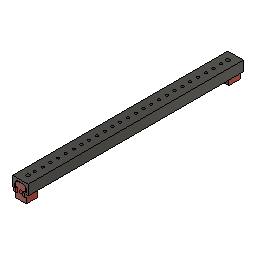
5_Assembly_Electro_support v5 (Autodesk Fusion 360 archive; units mm, degrees)
design "Support CI"
Autodesk Fusion 360 part; units mm, degrees
sketch "Sketch1" plane through (0, 0, 0) normal (0, 0, 1) x (1, 0, 0) in component "Support Electo"
  line L0 (138.5, -10) -> (-138.5, -10)
  line L1 (-138.5, -10) -> (-138.5, 10)
  line L2 (-138.5, 10) -> (138.5, 10)
  line L3 (138.5, 10) -> (138.5, -10)
  line L4 (138.5, -10) -> (-138.5, 10) construction
  line L5 (-138.5, -10) -> (138.5, 10) construction
  line L6 (138.5, -10) -> (138.5, 10)
  circle A0 centre (0, 0) radius 1.6
  circle A1 centre (-120, 0) radius 1.6
  circle A2 centre (-110, 0) radius 1.6
  circle A3 centre (-100, 0) radius 1.6
  circle A4 centre (-90, 0) radius 1.6
  circle A5 centre (-80, 0) radius 1.6
  circle A6 centre (-70, 0) radius 1.6
  circle A7 centre (-60, 0) radius 1.6
  circle A8 centre (-50, 0) radius 1.6
  circle A9 centre (-40, 0) radius 1.6
  circle A10 centre (-30, 0) radius 1.6
  circle A11 centre (-20, 0) radius 1.6
  circle A12 centre (-10, 0) radius 1.6
  circle A13 centre (10, 0) radius 1.6
  circle A14 centre (20, 0) radius 1.6
  circle A15 centre (30, 0) radius 1.6
  circle A16 centre (40, 0) radius 1.6
  circle A17 centre (50, 0) radius 1.6
  circle A18 centre (60, 0) radius 1.6
  circle A19 centre (70, 0) radius 1.6
  circle A20 centre (80, 0) radius 1.6
  circle A21 centre (90, 0) radius 1.6
  circle A22 centre (100, 0) radius 1.6
  circle A23 centre (110, 0) radius 1.6
  circle A24 centre (120, 0) radius 1.6
  line L7 (-138.5, 10) -> (138.5, 10)
  line L8 (138.5, 10) -> (138.5, 7)
  line L9 (138.5, 7) -> (-138.5, 7)
  line L10 (-138.5, 7) -> (-138.5, 10)
  line L11 (-138.5, -7) -> (138.5, -7)
  line L12 (138.5, -7) -> (138.5, -10)
  line L13 (138.5, -10) -> (-138.5, -10)
  line L14 (-138.5, -10) -> (-138.5, -7)
  line L15 (-138.5, -10) -> (-138.5, -7)
  line L16 (-138.5, 7) -> (-138.5, 10)
  circle A25 centre (-128.5, 0) radius 2.25
  circle A26 centre (128.5, 0) radius 2.25
  line L17 (-138.5, 0) -> (138.5, 0) construction
  dimension "d171" = 277
  dimension "d172" = 20
  dimension "d174" = 20
  dimension "d176" = 20
  dimension "d189" = 3.2
  dimension "d192" = 10
  dimension "d193" = 0
  dimension "d194" = 3
  dimension "d195" = 3
  dimension "d225" = 4.5
  dimension "d226" = 10
  dimension "d227" = 4.5
  dimension "d228" = 10
  constraint horizontal L0
  constraint perpendicular L0 L1
  constraint parallel L0 L2
  constraint parallel L1 L3
  constraint coincident L4 A0.centre
  constraint coincident L5 A0.centre
  constraint coincident A0.centre origin
  constraint vertical L15
  constraint vertical L6
  constraint horizontal L7
  constraint vertical L8
  constraint horizontal L9
  constraint vertical L10
  constraint coincident L3 L8.end
  constraint horizontal L11
  constraint vertical L12
  constraint horizontal L13
  constraint vertical L14
  constraint collinear L15 L16
  constraint midpoint L1 L17.start
  constraint midpoint L6 L17.end
  constraint coincident A26.centre L17
  constraint coincident A25.centre L17
  measures "d171" distance of L1.end L2.end
  measures "d172" distance of L0.end L1.end
  measures "d174" distance of L1.end L0.end
  measures "d176" distance of L2.end L0.start
  measures "d189" diameter of A0
  measures "d194" distance of L1.end L9.end
  measures "d195" distance of L11.start L0.end
  measures "d225" diameter of A25
  measures "d226" distance of L1 A25.centre
  measures "d227" diameter of A26
  measures "d228" distance of L6 A26.centre
extrude "Extrude6" add sketch "Sketch1" along normal blind 3 makes body 1 in component "Support Electo"
extrude "Extrude7" add sketch "Sketch1" against normal blind 10 contours L0 L1 L3 L6 L11 L12 L13 L14 L15 | L1 L2 L3 L6 L7 L8 L9 L10 L16 bodies 1 in component "Support Electo"
fillet "Fillet2" radius 4 2 edges at (0, 7, 0) (0, -7, 0) on bodies 1 in component "Support Electo"
sketch "Sketch1 (2)" plane through (0, 4.3249, 0) normal (0, -1, 0) x (1, 0, 0) in component "Equerre"
  line L0 (266.4871, 11.1429) -> (266.4871, 24.1429)
  line L1 (266.4871, 24.1429) -> (246.4871, 24.1429)
  line L2 (246.4871, 24.1429) -> (246.4871, 11.1429)
  line L3 (246.4871, 11.1429) -> (249.4871, 11.1429)
  line L4 (249.4871, 11.1429) -> (249.4871, 17.1429)
  arc A0 (253.4871, 21.1429) -> (249.4871, 17.1429) centre (253.4871, 17.1429) ccw
  line L5 (253.4871, 21.1429) -> (259.4871, 21.1429)
  arc A1 (263.4871, 17.1429) -> (259.4871, 21.1429) centre (259.4871, 17.1429) ccw
  line L6 (263.4871, 17.1429) -> (263.4871, 11.1429)
  line L7 (263.4871, 11.1429) -> (266.4871, 11.1429)
  arc A2 (263.4871, 17.1429) -> (259.4871, 21.1429) centre (259.4871, 17.1429) ccw
  line L8 (263.4871, 17.1429) -> (263.4871, 11.1429)
  line L9 (259.4871, 21.1429) -> (253.4871, 21.1429)
  arc A3 (253.4871, 21.1429) -> (249.4871, 17.1429) centre (253.4871, 17.1429) ccw
  line L10 (249.4871, 17.1429) -> (249.4871, 11.1429)
  line L11 (263.3871, 17.1429) -> (263.3871, 5.9705)
  line L12 (249.5871, 17.1429) -> (249.5871, 5.9705)
  arc A4 (253.4871, 21.0429) -> (249.5871, 17.1429) centre (253.4871, 17.1429) ccw
  line L13 (259.4871, 21.0429) -> (253.4871, 21.0429)
  arc A5 (263.3871, 17.1429) -> (259.4871, 21.0429) centre (259.4871, 17.1429) ccw
  line L14 (263.3871, 5.9705) -> (263.3871, 1.0429)
  line L15 (263.3871, 1.0429) -> (249.5871, 1.0429)
  line L16 (249.5871, 1.0429) -> (249.5871, 5.9705)
  line L17 (249.5871, 10.9429) -> (249.5871, 11.1429)
  line L18 (263.3871, 11.1429) -> (263.3871, 10.9429)
  line L19 (249.4871, 11.1429) -> (249.5871, 11.1429)
  circle A6 centre (256.4871, 11.0429) radius 2.1
  line L20 (249.5871, 11.0429) -> (263.3871, 11.0429) construction
  line L21 (263.3871, 8.0429) -> (249.5871, 8.0429)
  line L22 (249.5871, 8.0429) -> (249.5871, 14.0429)
  line L23 (249.5871, 14.0429) -> (263.3871, 14.0429)
  line L24 (263.3871, 14.0429) -> (263.3871, 8.0429)
  line L25 (263.3871, 8.0429) -> (249.5871, 14.0429) construction
  line L26 (249.5871, 8.0429) -> (263.3871, 14.0429) construction
  line L27 (260.9871, 8.0429) -> (251.9871, 8.0429)
  line L28 (251.9871, 8.0429) -> (251.9871, 14.0429)
  line L29 (251.9871, 14.0429) -> (260.9871, 14.0429)
  line L30 (260.9871, 14.0429) -> (260.9871, 8.0429)
  line L31 (260.9871, 8.0429) -> (251.9871, 14.0429) construction
  line L32 (251.9871, 8.0429) -> (260.9871, 14.0429) construction
  point P0 (256.4871, 11.0429)
  point P1 (256.4871, 11.0429)
  point P2 (256.4871, 11.0429)
  dimension "d268" = 4.2
  dimension "d273" = 20
  dimension "d274" = 0.1
  dimension "d275" = 10
  dimension "d276" = 6
  dimension "d282" = 9
  constraint coincident L3.end L4.start
  constraint vertical L14
  constraint horizontal L15
  constraint vertical L16
  constraint coincident L11.end L14.start
  constraint parallel L17 L18
  constraint coincident L14 L18.start
  constraint parallel L8 L11
  constraint parallel L10 L12
  constraint concentric A3 A4
  constraint parallel L9 L13
  constraint concentric A2 A5
  constraint tangent L13 A5
  constraint tangent L11 A5
  constraint tangent A4 L13
  constraint tangent L12 A4
  constraint coincident P2 P1
  constraint coincident L12 L20.start
  constraint coincident L11 L20.end
  constraint perpendicular L11 L20
  constraint coincident P2 L20
  constraint midpoint P2 L20
  constraint horizontal L21
  constraint perpendicular L21 L22
  constraint parallel L21 L23
  constraint parallel L22 L24
  constraint coincident L11 L21.start
  constraint coincident L25 P2
  constraint coincident L26 P2
  constraint horizontal L27
  constraint perpendicular L27 L28
  constraint parallel L27 L29
  constraint parallel L28 L30
  constraint coincident L31 P2
  constraint coincident L32 P2
  constraint coincident L21 L27.start
  measures "d268" diameter of A6
  measures "d273" distance of L13 L15
  measures "d274" distance of L4 L12
  measures "d275" distance of L15 L20
  measures "d276" distance of L21 L23
  measures "d282" distance of L28.end L29.end
extrude "Extrude1" add sketch "Sketch1 (2)" against normal blind 15 separate body contours L11 L12 A4 L13 A5 L23 L29 | L11 L18 L21 L23 L24 L30 | L21 L23 L27 L28 L29 L30 | L12 L17 L21 L22 L23 L28 | L11 L12 L14 L15 L16 L21 L27 makes body 2 in component "Equerre"
extrude "Extrude3" add sketch "Sketch1 (2)" along normal blind 2 contours L11 L18 L21 L23 L24 L30 | L12 L17 L21 L22 L23 L28 bodies 2 in component "Equerre"
sketch "Sketch2" plane through (0, 0, 21.1429) normal (0, 0, -1) x (1, 0, 0) in component "Equerre"
  line L0 (259.4871, -281.3249) -> (259.4871, -4.3249)
  line L1 (259.4871, -4.3249) -> (253.4871, -4.3249)
  line L2 (253.4871, -4.3249) -> (253.4871, -281.3249)
  line L3 (253.4871, -281.3249) -> (259.4871, -281.3249)
  circle A0 centre (256.4871, -142.8249) radius 1.6
  circle A1 centre (256.4871, -22.8249) radius 1.6
  circle A2 centre (256.4871, -32.8249) radius 1.6
  circle A3 centre (256.4871, -42.8249) radius 1.6
  circle A4 centre (256.4871, -52.8249) radius 1.6
  circle A5 centre (256.4871, -62.8249) radius 1.6
  circle A6 centre (256.4871, -72.8249) radius 1.6
  circle A7 centre (256.4871, -82.8249) radius 1.6
  circle A8 centre (256.4871, -92.8249) radius 1.6
  circle A9 centre (256.4871, -102.8249) radius 1.6
  circle A10 centre (256.4871, -112.8249) radius 1.6
  circle A11 centre (256.4871, -132.8249) radius 1.6
  circle A12 centre (256.4871, -122.8249) radius 1.6
  circle A13 centre (256.4871, -212.8249) radius 1.6
  circle A14 centre (256.4871, -202.8249) radius 1.6
  circle A15 centre (256.4871, -192.8249) radius 1.6
  circle A16 centre (256.4871, -182.8249) radius 1.6
  circle A17 centre (256.4871, -172.8249) radius 1.6
  circle A18 centre (256.4871, -162.8249) radius 1.6
  circle A19 centre (256.4871, -152.8249) radius 1.6
  circle A20 centre (256.4871, -271.3249) radius 2.25
  circle A21 centre (256.4871, -222.8249) radius 1.6
  circle A22 centre (256.4871, -232.8249) radius 1.6
  circle A23 centre (256.4871, -242.8249) radius 1.6
  circle A24 centre (256.4871, -252.8249) radius 1.6
  circle A25 centre (256.4871, -262.8249) radius 1.6
  circle A26 centre (256.4871, -14.4249) radius 0.75
  line L4 (256.4871, -4.3249) -> (256.4871, -14.4249) construction
  dimension "d277" = 1.5
  dimension "d279" = 10.1
  constraint midpoint L1 L4.start
  constraint coincident A26.centre L4.end
  constraint perpendicular L1 L4
  measures "d277" diameter of A26
  measures "d279" distance of L1 A26.centre
extrude "Extrude2" cut sketch "Sketch2" along normal blind 11 contours A26 bodies 2 in component "Equerre"
sketch "Sketch3" plane through (0, 19.3249, 0) normal (0, 1, 0) x (-1, 0, 0) in component "Equerre"
  circle A0 centre (-256.4871, 11.0429) radius 2.1
  line L0 (-263.3871, 17.1429) -> (-263.3871, 1.0429)
  line L1 (-263.3871, 1.0429) -> (-249.5871, 1.0429)
  line L2 (-249.5871, 1.0429) -> (-249.5871, 17.1429)
  arc A1 (-249.5871, 17.1429) -> (-253.4871, 21.0429) centre (-253.4871, 17.1429) ccw
  line L3 (-253.4871, 21.0429) -> (-259.4871, 21.0429)
  arc A2 (-259.4871, 21.0429) -> (-263.3871, 17.1429) centre (-259.4871, 17.1429) ccw
  circle A3 centre (-256.4871, 11.0429) radius 5
  dimension "d269" = 10
  constraint concentric A0 A3
  measures "d269" diameter of A3
extrude "Extrude4" cut sketch "Sketch3" against normal blind 8 contours A3 bodies 2 in component "Equerre"
chamfer "Chamfer1" distance 1.5 angle 45 2 edges at (262.1871, 2.3249, 8.0429) (250.7871, 2.3249, 8.0429) on bodies 2 in component "Equerre"
component "Support Electo" placed x (0, 1, 0) y (-1, 0, 0) z (0, 0, 1) at (230.1725, 147.8044, 52.437)
component "Equerre" placed x (1, 0, 0) y (0, 1, 0) z (0, 0, 1) at (-25.5646, 4.8794, 31.394)
component "Equerre" placed x (-1, 0, 0) y (0, -1, 0) z (0, 0, 1) at (485.9095, 290.7293, 31.394)
named bodies: "Equerre_Support_CI"

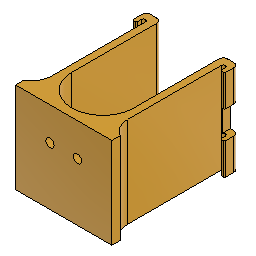
design "Support Batterie 5V"
Autodesk Fusion 360 part; units mm, degrees
sketch "Sketch1" plane through (0, 0, 0) normal (0, 0, 1) x (1, 0, 0)
  circle A0 centre (0, 0) radius 11.25
  line L0 (0, 0) -> (0, -12.75) construction
  line L1 (17.5, -14.25) -> (-17.5, -14.25)
  line L2 (-17.5, -14.25) -> (-17.5, -11.25)
  line L3 (-17.5, -11.25) -> (17.5, -11.25)
  line L4 (17.5, -11.25) -> (17.5, -14.25)
  line L5 (17.5, -14.25) -> (-17.5, -11.25) construction
  line L6 (-17.5, -14.25) -> (17.5, -11.25) construction
  line L7 (11.25, -11.25) -> (13.75, -11.25)
  line L8 (13.75, -11.25) -> (13.75, 29.3)
  line L9 (11.25, 30) -> (11.25, -11.25)
  line L10 (14.45, 30) -> (14.55, 30)
  line L11 (16.75, 30) -> (16.75, 30.9)
  line L12 (15.15, 32.5) -> (12.85, 32.5)
  line L13 (11.25, 30.9) -> (11.25, 30)
  line L14 (15.25, 29.3) -> (15.25, 28)
  line L15 (15.75, 27.5) -> (16.25, 27.5)
  line L16 (16.75, 28) -> (16.75, 30)
  arc A1 (14.45, 30) -> (13.75, 29.3) centre (14.45, 29.3) ccw
  arc A2 (15.25, 29.3) -> (14.55, 30) centre (14.55, 29.3) ccw
  arc A3 (15.25, 28) -> (15.75, 27.5) centre (15.75, 28) ccw
  arc A4 (16.25, 27.5) -> (16.75, 28) centre (16.25, 28) ccw
  arc A5 (16.75, 30.9) -> (15.15, 32.5) centre (15.15, 30.9) ccw
  arc A6 (12.85, 32.5) -> (11.25, 30.9) centre (12.85, 30.9) ccw
  arc A7 (-13.75, 29.3) -> (-14.45, 30) centre (-14.45, 29.3) ccw
  line L17 (-14.45, 30) -> (-14.55, 30)
  arc A8 (-14.55, 30) -> (-15.25, 29.3) centre (-14.55, 29.3) ccw
  line L18 (-15.25, 29.3) -> (-15.25, 28)
  arc A9 (-15.75, 27.5) -> (-15.25, 28) centre (-15.75, 28) ccw
  line L19 (-15.75, 27.5) -> (-16.25, 27.5)
  arc A10 (-16.75, 28) -> (-16.25, 27.5) centre (-16.25, 28) ccw
  line L20 (-16.75, 28) -> (-16.75, 30)
  line L21 (-16.75, 30) -> (-16.75, 30.9)
  arc A11 (-15.15, 32.5) -> (-16.75, 30.9) centre (-15.15, 30.9) ccw
  line L22 (-15.15, 32.5) -> (-12.85, 32.5)
  arc A12 (-11.25, 30.9) -> (-12.85, 32.5) centre (-12.85, 30.9) ccw
  line L23 (-11.25, 30.9) -> (-11.25, 30)
  line L24 (-11.25, 30) -> (-11.25, -11.25)
  line L25 (-11.25, -11.25) -> (-13.75, -11.25)
  line L26 (-13.75, -11.25) -> (-13.75, 29.3)
  point P0 (0, -12.75)
  point P1 (16.75, 32.5)
  point P2 (16.75, 27.5)
  dimension "d1" = 22.5
  dimension "d10" = 3
  dimension "d11" = 35
  dimension "d13" = 2.5
  dimension "d14" = 30
  dimension "d16" = 5.5
  dimension "d17" = 2.5
  dimension "d19" = 2.5
  dimension "d20" = 0.7
  dimension "d21" = 0.5
  dimension "d22" = 0.5
  dimension "d23" = 1.6
  dimension "d24" = 1.5
  constraint coincident A0.centre L0.start
  constraint horizontal L1
  constraint perpendicular L1 L2
  constraint parallel L1 L3
  constraint parallel L2 L4
  constraint coincident L5 P0
  constraint coincident L6 P0
  constraint coincident P0 L0.end
  constraint tangent A0 L3
  constraint vertical L0
  constraint horizontal L7
  constraint vertical L8
  constraint vertical L9
  constraint coincident L3 L7.start
  constraint tangent A0 L9
  constraint horizontal L10
  constraint vertical L11
  constraint horizontal L12
  constraint vertical L13
  constraint vertical L14
  constraint horizontal L15
  constraint vertical L16
  constraint coincident L9.start L10
  constraint tangent L8 A1
  constraint tangent L10 A1
  constraint coincident L11.start L10
  constraint tangent L10 A2
  constraint tangent L14 A2
  constraint equal A1 A2
  constraint tangent L14 A3
  constraint tangent L15 A3
  constraint coincident P2 L15
  constraint coincident P2 L16
  constraint tangent L15 A4
  constraint tangent L16 A4
  constraint coincident P1 L11
  constraint coincident P1 L12
  constraint tangent L11 A5
  constraint tangent L12 A5
  constraint tangent L12 A6
  constraint tangent L13 A6
  constraint equal A5 A6
  constraint symmetric L0 L7.start L24.end
  constraint symmetric L0 L7.end L25.end
  constraint symmetric L0 L9.start L23.end
  constraint symmetric L0 L11.start L20.end
  constraint symmetric L0 L8.end A7.start
  constraint symmetric L0 L10.start A7.end
  constraint symmetric L0 A1 A7
  constraint symmetric L0 L10.end L17.end
  constraint symmetric L0 L14.start A8.end
  constraint symmetric L0 A2 A8
  constraint symmetric L0 L14.end L18.end
  constraint symmetric L0 L15.start A9.start
  constraint symmetric L0 A3 A9
  constraint symmetric L0 L15.end L19.end
  constraint symmetric L0 L16.start A10.start
  constraint symmetric L0 A4 A10
  constraint symmetric L0 L11.end L21.end
  constraint symmetric L0 L12.start A11.start
  constraint symmetric L0 A5 A11
  constraint symmetric L0 L12.end L22.end
  constraint symmetric L0 L13.start A12.start
  constraint symmetric L0 A6 A12
  measures "d1" diameter of A0
  measures "d10" distance of L1.end L2.end
  measures "d11" distance of L1.start L1.end
  measures "d13" distance of L7.start L7.end
  measures "d14" vertical distance of A0.centre L9.start
  measures "d16" distance of L9.start L11.start
  measures "d17" distance of L11.start P1
  measures "d19" distance of L11.start P2
  measures "d20" radius of A1
  measures "d21" radius of A3
  measures "d22" radius of A4
  measures "d23" radius of A5
  measures "d24" distance of L14 L16
extrude "Extrude1" add sketch "Sketch1" along normal blind 30 contours A0 L3 L9 | L3 L7 L8 L9 L10 L11 L12 L13 L14 L15 L16 A1 A2 A3 A4 A5 A6 | L3 A7 L17 A8 L18 A9 L19 A10 L20 L21 A11 L22 A12 L23 L24 L25 L26 | A0 L3 L24 | L1 L2 L3 L4 L7 L25
fillet "Fillet1" radius 7.5 2 edges at (-13.75, -11.25, 15) (13.75, -11.25, 15)
sketch "Sketch2" plane through (0, -14.25, 0) normal (0, -1, 0) x (1, 0, 0)
  line L0 (-17.5, 0) -> (17.5, 0)
  line L1 (17.5, 0) -> (17.5, 30)
  line L2 (17.5, 30) -> (-17.5, 30)
  line L3 (-17.5, 30) -> (-17.5, 0)
  line L4 (0, 0) -> (0, 18) construction
  line L5 (-5, 18) -> (5, 18)
  circle A0 centre (-5, 18) radius 1.5
  circle A1 centre (5, 18) radius 1.5
  dimension "d29" = 18
  dimension "d30" = 10
  dimension "d31" = 3
  dimension "d32" = 3
  constraint coincident L4.start origin
  constraint perpendicular L0 L4
  constraint perpendicular L4 L5
  constraint coincident L4.end L5
  constraint midpoint L4.end L5
  constraint coincident L5.start A0.centre
  constraint coincident L5.end A1.centre
  measures "d29" distance of L4.start L4.end
  measures "d30" distance of L5.start L5.end
  measures "d31" diameter of A0
  measures "d32" diameter of A1
extrude "Extrude2" cut sketch "Sketch2" against normal through all contours A0 | A1
ref_plane "WorkPlane1" through (0, -11.25, 15) normal (0, -1, 0) x (1, 0, 0)
sketch "Sketch4" plane through (0, -11.25, 15) normal (0, -1, 0) x (1, 0, 0)
  circle A0 centre (-5, 3) radius 1.5
  circle A1 centre (5, 3) radius 1.5
  circle A2 centre (-5, 3) radius 3
  circle A3 centre (5, 3) radius 3
  dimension "d38" = 6
  dimension "d39" = 6
  constraint concentric A0 A2
  constraint concentric A1 A3
  measures "d38" diameter of A2
  measures "d39" diameter of A3
extrude "Extrude4" cut sketch "Sketch4" against normal blind 14
sketch "Sketch5" plane through (0, 0, 0) normal (0, 0, -1) x (1, 0, 0)
  arc A0 (17.5, 11.25) -> (13.75, 4.7548) centre (21.25, 4.7548) ccw
  line L0 (17.5, 11.25) -> (17.5, 14.25)
  line L1 (17.5, 14.25) -> (-17.5, 14.25)
  line L2 (-17.5, 14.25) -> (-17.5, 11.25)
  arc A1 (-13.75, 4.7548) -> (-17.5, 11.25) centre (-21.25, 4.7548) ccw
  line L3 (-13.75, 4.7548) -> (-13.75, -29.3)
  arc A2 (-14.45, -30) -> (-13.75, -29.3) centre (-14.45, -29.3) ccw
  line L4 (-14.45, -30) -> (-14.55, -30)
  arc A3 (-15.25, -29.3) -> (-14.55, -30) centre (-14.55, -29.3) ccw
  line L5 (-15.25, -29.3) -> (-15.25, -28)
  arc A4 (-15.25, -28) -> (-15.75, -27.5) centre (-15.75, -28) ccw
  line L6 (-15.75, -27.5) -> (-16.25, -27.5)
  arc A5 (-16.25, -27.5) -> (-16.75, -28) centre (-16.25, -28) ccw
  line L7 (-16.75, -28) -> (-16.75, -30.9)
  arc A6 (-16.75, -30.9) -> (-15.15, -32.5) centre (-15.15, -30.9) ccw
  line L8 (-15.15, -32.5) -> (-12.85, -32.5)
  arc A7 (-12.85, -32.5) -> (-11.25, -30.9) centre (-12.85, -30.9) ccw
  line L9 (-11.25, -30.9) -> (-11.25, 0)
  arc A8 (11.25, 0) -> (-11.25, 0) centre (0, 0) ccw
  line L10 (11.25, 0) -> (11.25, -30.9)
  arc A9 (11.25, -30.9) -> (12.85, -32.5) centre (12.85, -30.9) ccw
  line L11 (12.85, -32.5) -> (15.15, -32.5)
  arc A10 (15.15, -32.5) -> (16.75, -30.9) centre (15.15, -30.9) ccw
  line L12 (16.75, -30.9) -> (16.75, -28)
  arc A11 (16.75, -28) -> (16.25, -27.5) centre (16.25, -28) ccw
  line L13 (16.25, -27.5) -> (15.75, -27.5)
  arc A12 (15.75, -27.5) -> (15.25, -28) centre (15.75, -28) ccw
  line L14 (15.25, -28) -> (15.25, -29.3)
  arc A13 (14.55, -30) -> (15.25, -29.3) centre (14.55, -29.3) ccw
  line L15 (14.55, -30) -> (14.45, -30)
  arc A14 (13.75, -29.3) -> (14.45, -30) centre (14.45, -29.3) ccw
  line L16 (13.75, -29.3) -> (13.75, 4.7548)
  line L17 (-11.25, 0) -> (11.25, 0)
  constraint coincident L9.end A8.end
  constraint coincident A8.start L10.start
extrude "Extrude5" add sketch "Sketch5" along normal blind 3
sketch "Sketch6" plane through (0, 32.5, 0) normal (0, 1, 0) x (-1, 0, 0)
  line L0 (15.15, -3) -> (15.15, 30)
  line L1 (15.15, 30) -> (12.85, 30)
  line L2 (12.85, 30) -> (12.85, -3)
  line L3 (12.85, -3) -> (15.15, -3)
  line L4 (-12.85, -3) -> (-12.85, 30)
  line L5 (-12.85, 30) -> (-15.15, 30)
  line L6 (-15.15, 30) -> (-15.15, -3)
  line L7 (-15.15, -3) -> (-12.85, -3)
  line L8 (-15.15, 18.5) -> (-22.1698, 18.5)
  line L9 (-22.1698, 18.5) -> (-22.1698, 8.5)
  line L10 (-22.1698, 8.5) -> (-15.15, 8.5)
  line L11 (-15.15, 8.5) -> (-15.15, 18.5)
  line L12 (15.15, 18.5) -> (21.4643, 18.5)
  line L13 (21.4643, 18.5) -> (21.4643, 8.5)
  line L14 (21.4643, 8.5) -> (15.15, 8.5)
  line L15 (15.15, 8.5) -> (15.15, 18.5)
  line L16 (15.15, 18.5) -> (13.85, 18.5)
  line L17 (13.85, 18.5) -> (13.85, 8.5)
  line L18 (13.85, 8.5) -> (15.15, 8.5)
  line L19 (15.15, 8.5) -> (15.15, 18.5)
  line L20 (-15.15, 18.5) -> (-13.85, 18.5)
  line L21 (-13.85, 18.5) -> (-13.85, 8.5)
  line L22 (-13.85, 8.5) -> (-15.15, 8.5)
  line L23 (-15.15, 8.5) -> (-15.15, 18.5)
  dimension "d44" = 10
  dimension "d45" = 10
  dimension "d48" = 1.3
  dimension "d49" = 1.3
  constraint horizontal L8
  constraint vertical L9
  constraint horizontal L10
  constraint vertical L11
  constraint coincident L6 L8.start
  constraint horizontal L12
  constraint vertical L13
  constraint horizontal L14
  constraint vertical L15
  constraint coincident L0 L12.start
  constraint midpoint L6 L11
  constraint midpoint L0 L15
  constraint horizontal L16
  constraint vertical L17
  constraint horizontal L18
  constraint vertical L19
  constraint coincident L14.end L15.start
  constraint horizontal L20
  constraint vertical L21
  constraint horizontal L22
  constraint vertical L23
  constraint coincident L10.end L11.start
  measures "d44" distance of L8.start L10.end
  measures "d45" distance of L12.start L14.end
  measures "d48" distance of L12.start L16.end
  measures "d49" distance of L8.start L20.end
extrude "Extrude6" cut sketch "Sketch6" against normal blind 9 contours L0 L15 L16 L17 L18 L19 | L0 L12 L13 L14 L15 L19 | L6 L8 L9 L10 L11 L23 | L6 L11 L20 L21 L22 L23
named bodies: "Support_Bat5V"

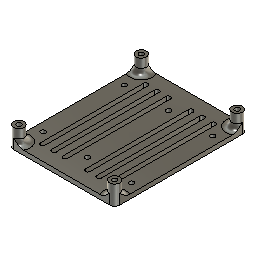
design "Support CI"
Autodesk Fusion 360 part; units mm, degrees
sketch "Sketch1" plane through (0, 0, 0) normal (0, 0, 1) x (1, 0, 0)
  line L0 (32.5, -45) -> (-32.5, -45)
  line L1 (-36, -41.5) -> (-36, 41.5)
  line L2 (-32.5, 45) -> (32.5, 45)
  line L3 (36, 41.5) -> (36, -41.5)
  line L4 (36, -45) -> (-36, 45) construction
  line L5 (-36, -45) -> (36, 45) construction
  line L6 (32.5, -41.5) -> (-32.5, -41.5) construction
  line L7 (-32.5, -41.5) -> (-32.5, 41.5) construction
  line L8 (-32.5, 41.5) -> (32.5, 41.5) construction
  line L9 (32.5, 41.5) -> (32.5, -41.5) construction
  line L10 (32.5, -41.5) -> (-32.5, 41.5) construction
  line L11 (-32.5, -41.5) -> (32.5, 41.5) construction
  circle A0 centre (-32.5, 41.5) radius 3.5
  circle A1 centre (32.5, 41.5) radius 3.5
  circle A2 centre (-32.5, -41.5) radius 3.5
  circle A3 centre (32.5, -41.5) radius 3.5
  circle A4 centre (-32.5, 41.5) radius 1.6
  circle A5 centre (32.5, 41.5) radius 1.6
  circle A6 centre (32.5, -41.5) radius 1.6
  circle A7 centre (-32.5, -41.5) radius 1.6
  arc A8 (-32.5, 45) -> (-36, 41.5) centre (-32.5, 41.5) ccw
  arc A9 (36, 41.5) -> (32.5, 45) centre (32.5, 41.5) ccw
  arc A10 (32.5, -45) -> (36, -41.5) centre (32.5, -41.5) ccw
  arc A11 (-36, -41.5) -> (-32.5, -45) centre (-32.5, -41.5) ccw
  line L12 (30, -27.5) -> (-30, -27.5) construction
  line L13 (-30, -27.5) -> (-30, 27.5) construction
  line L14 (-30, 27.5) -> (30, 27.5) construction
  line L15 (30, 27.5) -> (30, -27.5) construction
  line L16 (30, -27.5) -> (-30, 27.5) construction
  line L17 (-30, -27.5) -> (30, 27.5) construction
  circle A12 centre (-30, 27.5) radius 1.6
  circle A13 centre (0, 27.5) radius 1.6
  circle A14 centre (30, 27.5) radius 1.6
  circle A15 centre (-30, -27.5) radius 1.6
  circle A16 centre (0, -27.5) radius 1.6
  circle A17 centre (30, -27.5) radius 1.6
  line L18 (-1.5, 35) -> (-1.5, -35)
  arc A18 (-1.5, -35) -> (1.5, -35) centre (0, -35) ccw
  line L19 (1.5, -35) -> (1.5, 35)
  arc A19 (1.5, 35) -> (-1.5, 35) centre (0, 35) ccw
  line L20 (0, 35) -> (0, -35) construction
  line L21 (-24.5, 35) -> (-24.5, -35)
  arc A20 (-24.5, -35) -> (-21.5, -35) centre (-23, -35) ccw
  line L22 (-21.5, -35) -> (-21.5, 35)
  arc A21 (-21.5, 35) -> (-24.5, 35) centre (-23, 35) ccw
  line L23 (-16.8333, 35) -> (-16.8333, -35)
  arc A22 (-16.8333, -35) -> (-13.8333, -35) centre (-15.3333, -35) ccw
  line L24 (-13.8333, -35) -> (-13.8333, 35)
  arc A23 (-13.8333, 35) -> (-16.8333, 35) centre (-15.3333, 35) ccw
  line L25 (-9.1667, 35) -> (-9.1667, -35)
  arc A24 (-9.1667, -35) -> (-6.1667, -35) centre (-7.6667, -35) ccw
  line L26 (-6.1667, -35) -> (-6.1667, 35)
  arc A25 (-6.1667, 35) -> (-9.1667, 35) centre (-7.6667, 35) ccw
  line L27 (6.1667, 35) -> (6.1667, -35)
  arc A26 (6.1667, -35) -> (9.1667, -35) centre (7.6667, -35) ccw
  line L28 (9.1667, -35) -> (9.1667, 35)
  arc A27 (9.1667, 35) -> (6.1667, 35) centre (7.6667, 35) ccw
  line L29 (13.8333, 35) -> (13.8333, -35)
  arc A28 (13.8333, -35) -> (16.8333, -35) centre (15.3333, -35) ccw
  line L30 (16.8333, -35) -> (16.8333, 35)
  arc A29 (16.8333, 35) -> (13.8333, 35) centre (15.3333, 35) ccw
  line L31 (21.5, 35) -> (21.5, -35)
  arc A30 (21.5, -35) -> (24.5, -35) centre (23, -35) ccw
  line L32 (24.5, -35) -> (24.5, 35)
  arc A31 (24.5, 35) -> (21.5, 35) centre (23, 35) ccw
  dimension "d1" = 72
  dimension "d2" = 90
  dimension "d3" = 65
  dimension "d4" = 83
  dimension "d5" = 7
  dimension "d6" = 7
  dimension "d7" = 7
  dimension "d8" = 7
  dimension "d9" = 3.2
  dimension "d10" = 3.2
  dimension "d11" = 3.2
  dimension "d12" = 3.2
  dimension "d13" = 3.5
  dimension "d14" = 60
  dimension "d15" = 55
  dimension "d16" = 3.2
  dimension "d17" = 3.2
  dimension "d18" = 3.2
  dimension "d19" = 3.2
  dimension "d20" = 3.2
  dimension "d21" = 3.2
  dimension "d22" = 3
  dimension "d25" = 23
  dimension "d26" = 0
  dimension "d27" = 70
  constraint horizontal L0
  constraint perpendicular L0 L1
  constraint parallel L0 L2
  constraint parallel L1 L3
  constraint coincident L4 origin
  constraint coincident L5 origin
  constraint horizontal L6
  constraint perpendicular L6 L7
  constraint parallel L6 L8
  constraint parallel L7 L9
  constraint coincident L10 origin
  constraint coincident L11 origin
  constraint coincident L7.end L8.start
  constraint coincident L8.end L9.start
  constraint coincident L6.end L7.start
  constraint coincident L6.start L9.end
  constraint concentric A0 A4
  constraint concentric A3 A6
  constraint concentric A2 A7
  constraint coincident L4.end L2
  constraint coincident L4.end L1
  constraint tangent L2 A8
  constraint tangent L1 A8
  constraint coincident L5.end L2
  constraint coincident L5.end L3
  constraint tangent L2 A9
  constraint tangent L3 A9
  constraint equal A8 A9
  constraint coincident L4.start L3
  constraint coincident L4.start L0
  constraint tangent L3 A10
  constraint tangent L0 A10
  constraint equal A8 A10
  constraint coincident L5.start L0
  constraint coincident L5.start L1
  constraint tangent L0 A11
  constraint tangent L1 A11
  constraint equal A8 A11
  constraint horizontal L12
  constraint perpendicular L12 L13
  constraint parallel L12 L14
  constraint parallel L13 L15
  constraint coincident L16 origin
  constraint coincident L17 origin
  constraint coincident L13.end L14.start
  constraint midpoint L14 A13.centre
  constraint coincident L14.end L15.start
  constraint coincident L12.end L13.start
  constraint midpoint L12 A16.centre
  constraint coincident L12.start L15.end
  constraint tangent L18 A18
  constraint tangent A18 L19
  constraint parallel L18 L19
  constraint tangent L19 A19
  constraint tangent L18 A19
  constraint vertical L20
  constraint midpoint L20 origin
  measures "d1" distance of L4.end L5.end
  measures "d2" distance of L5.start L4.end
  measures "d3" distance of L7.end L8.end
  measures "d4" distance of L6.end L7.end
  measures "d5" diameter of A0
  measures "d6" diameter of A1
  measures "d7" diameter of A2
  measures "d8" diameter of A3
  measures "d9" diameter of A4
  measures "d10" diameter of A5
  measures "d11" diameter of A6
  measures "d12" diameter of A7
  measures "d13" radius of A8
  measures "d14" distance of L13.end L14.end
  measures "d15" distance of L12.end L13.end
  measures "d16" diameter of A12
  measures "d17" diameter of A13
  measures "d18" diameter of A14
  measures "d19" diameter of A15
  measures "d20" diameter of A16
  measures "d21" diameter of A17
  measures "d22" diameter of A18
  measures "d27" distance of A19.centre A18.centre
extrude "Extrude1" add sketch "Sketch1" against normal blind 3 contours L0 L1 L2 L3 A0 A1 A2 A3 | A3 A10 | A2 A11 | A1 A9 | A0 A8 | A13 L18 L19 A19 | A13 A16 L18 L19 | A16 L18 A18 L19
extrude "Extrude2" add sketch "Sketch1" along normal blind 10 contours A3 A10 | A2 A11 | A1 A9 | A0 A8
fillet "Fillet1" radius 4 4 edges at (-30.0251, -39.0251, 0) (-30.0251, 39.0251, 0) (30.0251, 39.0251, 0) (30.0251, -39.0251, 0)

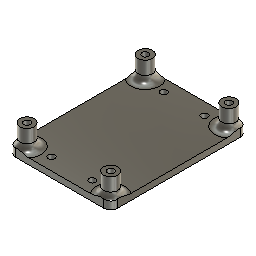
design "Support Alim DC-DC"
Autodesk Fusion 360 part; units mm, degrees
sketch "Sketch1" plane through (0, 0, 0) normal (0, 0, 1) x (1, 0, 0)
  line L0 (21.5, -33.5) -> (-21.5, -33.5)
  line L1 (-25, -30) -> (-25, 30)
  line L2 (-21.5, 33.5) -> (21.5, 33.5)
  line L3 (25, 30) -> (25, -30)
  line L4 (25, -33.5) -> (-25, 33.5) construction
  line L5 (-25, -33.5) -> (25, 33.5) construction
  line L6 (20.5, -29) -> (-20.5, -29) construction
  line L7 (-20.5, -29) -> (-20.5, 29) construction
  line L8 (-20.5, 29) -> (20.5, 29) construction
  line L9 (20.5, 29) -> (20.5, -29) construction
  line L10 (20.5, -29) -> (-20.5, 29) construction
  line L11 (-20.5, -29) -> (20.5, 29) construction
  circle A0 centre (-20.5, 29) radius 3.5
  circle A1 centre (20.5, 29) radius 3.5
  circle A2 centre (-20.5, -29) radius 3.5
  circle A3 centre (20.5, -29) radius 3.5
  circle A4 centre (-20.5, 29) radius 1.6
  circle A5 centre (20.5, 29) radius 1.6
  circle A6 centre (20.5, -29) radius 1.6
  circle A7 centre (-20.5, -29) radius 1.6
  arc A8 (-21.5, 33.5) -> (-25, 30) centre (-21.5, 30) ccw
  arc A9 (25, 30) -> (21.5, 33.5) centre (21.5, 30) ccw
  arc A10 (21.5, -33.5) -> (25, -30) centre (21.5, -30) ccw
  arc A11 (-25, -30) -> (-21.5, -33.5) centre (-21.5, -30) ccw
  line L12 (10, -27.5) -> (-10, -27.5) construction
  line L13 (-10, -27.5) -> (-10, 27.5) construction
  line L14 (-10, 27.5) -> (10, 27.5) construction
  line L15 (10, 27.5) -> (10, -27.5) construction
  line L16 (10, -27.5) -> (-10, 27.5) construction
  line L17 (-10, -27.5) -> (10, 27.5) construction
  circle A12 centre (-10, 27.5) radius 1.6
  circle A13 centre (10, 27.5) radius 1.6
  circle A14 centre (-10, -27.5) radius 1.6
  circle A15 centre (10, -27.5) radius 1.6
  line L18 (0, 33.5) -> (0, -33.5) construction
  dimension "d1" = 50
  dimension "d2" = 67
  dimension "d3" = 41
  dimension "d4" = 58
  dimension "d5" = 7
  dimension "d6" = 7
  dimension "d7" = 7
  dimension "d8" = 7
  dimension "d9" = 3.2
  dimension "d10" = 3.2
  dimension "d11" = 3.2
  dimension "d12" = 3.2
  dimension "d13" = 3.5
  dimension "d14" = 20
  dimension "d15" = 55
  dimension "d16" = 3.2
  dimension "d18" = 3.2
  dimension "d19" = 3.2
  dimension "d21" = 3.2
  constraint horizontal L0
  constraint perpendicular L0 L1
  constraint parallel L0 L2
  constraint parallel L1 L3
  constraint coincident L4 origin
  constraint coincident L5 origin
  constraint horizontal L6
  constraint perpendicular L6 L7
  constraint parallel L6 L8
  constraint parallel L7 L9
  constraint coincident L10 origin
  constraint coincident L11 origin
  constraint coincident L7.end L8.start
  constraint coincident L8.end L9.start
  constraint coincident L6.end L7.start
  constraint coincident L6.start L9.end
  constraint concentric A0 A4
  constraint concentric A3 A6
  constraint concentric A2 A7
  constraint coincident L4.end L2
  constraint coincident L4.end L1
  constraint tangent L2 A8
  constraint tangent L1 A8
  constraint coincident L5.end L2
  constraint coincident L5.end L3
  constraint tangent L2 A9
  constraint tangent L3 A9
  constraint equal A8 A9
  constraint coincident L4.start L3
  constraint coincident L4.start L0
  constraint tangent L3 A10
  constraint tangent L0 A10
  constraint equal A8 A10
  constraint coincident L5.start L0
  constraint coincident L5.start L1
  constraint tangent L0 A11
  constraint tangent L1 A11
  constraint equal A8 A11
  constraint horizontal L12
  constraint perpendicular L12 L13
  constraint parallel L12 L14
  constraint parallel L13 L15
  constraint coincident L16 origin
  constraint coincident L17 origin
  constraint coincident L13.end L14.start
  constraint coincident L14.end L15.start
  constraint coincident L12.end L13.start
  constraint coincident L12.start L15.end
  constraint vertical L18
  constraint midpoint L18 origin
  constraint coincident L2 L18.start
  measures "d1" distance of L4.end L5.end
  measures "d2" distance of L5.start L4.end
  measures "d3" distance of L7.end L8.end
  measures "d4" distance of L6.end L7.end
  measures "d5" diameter of A0
  measures "d6" diameter of A1
  measures "d7" diameter of A2
  measures "d8" diameter of A3
  measures "d9" diameter of A4
  measures "d10" diameter of A5
  measures "d11" diameter of A6
  measures "d12" diameter of A7
  measures "d13" radius of A8
  measures "d14" distance of L13.end L14.end
  measures "d15" distance of L12.end L13.end
  measures "d16" diameter of A12
  measures "d18" diameter of A13
  measures "d19" diameter of A14
  measures "d21" diameter of A15
extrude "Extrude1" add sketch "Sketch1" against normal blind 3 contours L0 L1 L2 L3 A8 A9 A10 A11 | A0 | A1 | A2 | A3
extrude "Extrude2" add sketch "Sketch1" along normal blind 10 contours A0 | A1 | A2 | A3
sketch "Sketch2" plane through (0, 0, -3) normal (0, 0, -1) x (1, 0, 0)
  circle A0 centre (-20.5, 29) radius 1.6
  circle A1 centre (-20.5, -29) radius 1.6
  circle A2 centre (10, 27.5) radius 1.6
  circle A3 centre (-10, -27.5) radius 1.6
  circle A4 centre (-10, 27.5) radius 1.6
  circle A5 centre (10, -27.5) radius 1.6
  arc A6 (-25, -30) -> (-21.5, -33.5) centre (-20.5, -29) ccw
  line L0 (-21.5, -33.5) -> (21.5, -33.5)
  arc A7 (21.5, -33.5) -> (25, -30) centre (21.5, -30) ccw
  line L1 (25, -30) -> (25, 30)
  arc A8 (25, 30) -> (21.5, 33.5) centre (21.5, 30) ccw
  line L2 (21.5, 33.5) -> (-21.5, 33.5)
  arc A9 (-21.5, 33.5) -> (-25, 30) centre (-20.5, 29) ccw
  line L3 (-25, 30) -> (-25, -30)
  circle A10 centre (-20.5, 29) radius 3
  circle A11 centre (-20.5, -29) radius 3
  circle A12 centre (20.5, 29) radius 3
  circle A13 centre (20.5, -29) radius 3
  point P0 (-21.5, -30)
  point P1 (-21.5, 30)
  point P2 (20.5, -29)
  point P3 (20.5, 29)
  point P4 (-21.5, -30)
  point P5 (-21.5, 30)
  point P6 (20.5, -29)
  point P7 (20.5, 29)
  point P8 (-21.5, -30)
  point P9 (-21.5, 30)
  dimension "d33" = 6
  dimension "d35" = 6
  dimension "d40" = 6
  dimension "d41" = 6
  constraint concentric A0 A10
  constraint concentric A1 A11
  constraint coincident P7 P3
  constraint coincident P6 P2
  measures "d33" diameter of A10
  measures "d35" diameter of A11
  measures "d40" diameter of A12
  measures "d41" diameter of A13
extrude "Extrude3" cut sketch "Sketch2" against normal blind 2.5 contours A10 | A11 | A12 | A13
fillet "Fillet2" radius 3.5 4 edges at (-23.7631, -27.7343, 0) (-23.7631, 30.2657, 0) (17.2369, 30.2657, 0) (17.2369, -27.7343, 0)
